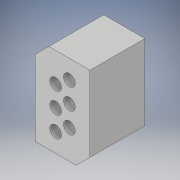
# Autodesk Inventor part: con_case
Saved by Autodesk Inventor 2019 (Build 230136000, 136)
## iProperties
Created: 2018-10-20
Part Number: con_case
Material: Generisch
Document SubType Name: Modeling
Designer: WhoTheHeck
Density: 1 g/cm^3
Appearance: Vorgabe
Author: WhoTheHeck
Autodesk Inventor part; units mm, degrees
ref_plane "YZ Plane" through (0, 0, 0) normal (1, 0, 0) x (0, 1, 0)
ref_plane "XZ Plane" through (0, 0, 0) normal (0, 1, 0) x (-1, 0, 0)
ref_plane "XY Plane" through (0, 0, 0) normal (0, 0, 1) x (1, 0, 0)
sketch "Skizze1" plane through (0, 0, 0) normal (0, 0, 1) x (1, 0, 0)
  circle A0 centre (0, 0) radius 0.85
  line L0 (0, 0) -> (2, 0) construction
  line L1 (2, 0) -> (2, 1.5) construction
  line L2 (0, 0) -> (0, 3) construction
  circle A1 centre (0, 3) radius 0.85
  circle A2 centre (2, 1.5) radius 0.85
  circle A3 centre (0, 6) radius 0.85
  circle A4 centre (2, 4.5) radius 0.85
  circle A5 centre (2, 7.5) radius 0.85
  line L3 (2, 7.5) -> (2, 4.5) construction
  line L4 (2, 4.5) -> (2, 1.5) construction
  line L5 (0, 3) -> (0, 6) construction
  line L6 (-3, 10.25) -> (5, 10.25)
  line L7 (5, 10.25) -> (5, -2.75)
  line L8 (5, -2.75) -> (-3, -2.75)
  line L9 (-3, -2.75) -> (-3, 10.25)
  dimension "d0" = 1.7
  dimension "d1" = 2
  dimension "d2" = 1.5
  dimension "d3" = 3
  dimension "d4" = 1.7
  dimension "d5" = 1.7
  dimension "d6" = 1.7
  dimension "d7" = 1.7
  dimension "d8" = 1.7
  dimension "d9" = 3
  dimension "d10" = 3
  dimension "d11" = 3
  dimension "d23" = 8
  dimension "d24" = 2
  dimension "d25" = 3
  dimension "d26" = 13
  dimension "d27" = 7.5
  dimension "d28" = 2.75
  constraints: 20 end point, 6 centre point, 3 coincident, 3 equal length, 3 vertical, 2 horizontal, 2 perpendicular
  measures "d0" diameter of A0
  measures "d1" distance of L0.start L0.end
  measures "d2" distance of L0.end L1.end
  measures "d3" distance of L0.start L2.end
  measures "d4" diameter of A1
  measures "d5" diameter of A2
  measures "d6" diameter of A3
  measures "d7" diameter of A4
  measures "d8" diameter of A5
  measures "d9" distance of L5.end L2.end
  measures "d10" distance of L3.end L1.end
  measures "d11" distance of L3.start L3.end
  measures "d23" distance of L7.end L8.end
  measures "d24" distance between parallel lines of L4 L5
  measures "d25" distance between parallel lines of L5 L9
  measures "d26" distance of L8.end L6.start
  measures "d27" vertical distance of point (0, 0) L3.start
  measures "d28" distance from line of L3.start L6
extrude "Extrusion1" add sketch "Skizze1" along normal blind 8
chamfer "Fase1" distance 2 angle 45 2 edges at (5, -2.75, 4) (-3, 10.25, 4)
sketch "Skizze2" plane through (-3, -2.75, 0) normal (-1, 0, 0) x (0, 0, 1)
  line L0 (2.2899, 8.4375) -> (7.9071, 8.4375) construction
  line L1 (7.9071, 8.4375) -> (7.9071, -0.4674) construction
  line L2 (7.9071, -0.4674) -> (2.2899, -0.4674) construction
  line L3 (2.2899, -0.4674) -> (2.2899, 8.4375) construction
  point P0 (0, 2.75)
  constraints: 2 other
extrude "Extrusion2" [suppressed]
equation "\"d4\" = d0"
equation "\"d5\" = d4"
equation "\"d6\" = d4"
equation "\"d7\" = d4"
equation "\"d8\" = d6"
equation "\"d9\" = d3"
equation "\"d10\" = d3"
equation "\"d11\" = d3"
